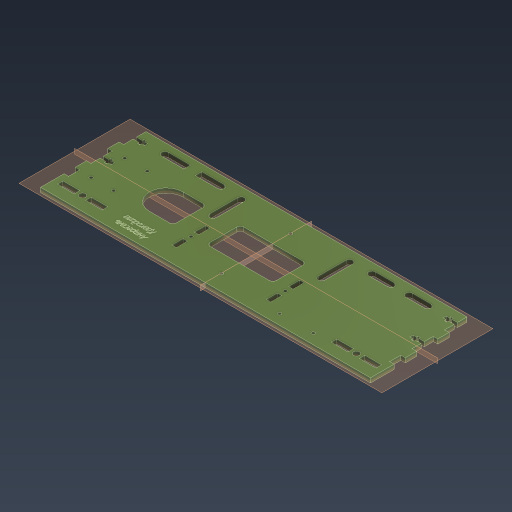
# Autodesk Inventor part: Фанерка_аккумуляторов
Saved by Autodesk Inventor 2023.2 (Build 272271030, 271C)
## iProperties
Created: 2025-12-29
Part Number: Фанерка_аккумуляторов
Material: Типовые
Document SubType Name: Modeling
Designer: Олег Коноваленко
Density: 1 g/cm^3
Appearance: Темно-оливковый
Author: Олег Коноваленко
Autodesk Inventor part; units mm, degrees
sketch "Эскиз1" plane through (0, 0, 0) normal (0, 1, 0) x (-1, 0, 0)
  line L0 (147, 45) -> (-147, 45)
  line L1 (-147, 45) -> (-147, -45)
  line L2 (-147, -45) -> (147, -45)
  line L3 (147, -45) -> (147, 45)
  line L4 (147, 45) -> (-147, -45) construction
  line L5 (-147, 45) -> (147, -45) construction
  point P0 (0, 0)
  dimension "d3" = 294
  dimension "d4" = 90
  constraints: 12 end point, 2 midpoint, 2 parallel, 1 horizontal, 1 perpendicular
  measures "d3" distance of L1.end L2.end
  measures "d4" distance of L0.end L1.end
extrude "Выдавливание1" add sketch "Эскиз1" along normal mid plane 4
sketch "Эскиз2" plane through (0, 2, 0) normal (0, 1, 0) x (1, 0, 0)
  line L0 (-127, -35) -> (-127, -30) projected
  line L1 (-127, -30) -> (-142, -30) projected
  line L2 (-142, -30) -> (-142, -35) projected
  line L3 (-142, -35) -> (-127, -35) projected
  line L4 (-102, -35) -> (-102, -30) projected
  line L5 (-102, -30) -> (-117, -30) projected
  line L6 (-117, -30) -> (-117, -35) projected
  line L7 (-117, -35) -> (-102, -35) projected
  line L8 (102, -35) -> (102, -30) projected
  line L9 (117, -35) -> (102, -35) projected
  line L10 (117, -30) -> (117, -35) projected
  line L11 (102, -30) -> (117, -30) projected
  line L12 (127, -35) -> (127, -30) projected
  line L13 (142, -35) -> (127, -35) projected
  line L14 (142, -30) -> (142, -35) projected
  line L15 (127, -30) -> (142, -30) projected
  circle A0 centre (122, -32.5) radius 2.8 projected
  circle A1 centre (-122, -32.5) radius 2.8 projected
  point P0 (0, 0)
extrude "Выдавливание2" cut sketch "Эскиз2" against normal up to next
sketch "Эскиз3" plane through (0, 2, 0) normal (0, 1, 0) x (1, 0, 0)
  line L0 (80, 0) -> (-80, 0) construction
  line L1 (80, 15) -> (-80, 15)
  line L2 (-80, -15) -> (80, -15)
  arc A0 (80, -15) -> (80, 15) centre (80, 0) ccw
  arc A1 (-80, 15) -> (-80, -15) centre (-80, 0) ccw
  line L3 (55, -15) -> (30, -15)
  line L4 (30, -15) -> (30, 15)
  line L5 (30, 15) -> (55, 15)
  line L6 (55, 15) -> (55, -15)
  line L7 (-29, -15) -> (-59, -15)
  line L8 (-59, -15) -> (-59, 15)
  line L9 (-59, 15) -> (-29, 15)
  line L10 (-29, 15) -> (-29, -15)
  line L11 (-44, -11) -> (-44, -1) projected
  line L12 (40, -11) -> (40, -1) projected
  point P0 (0, 0)
  point P1 (-29, 15)
  dimension "d7" = 160
  dimension "d8" = 15
  dimension "d11" = 25
  dimension "d12" = 30
  dimension "d13" = 10
  dimension "d14" = 15
  constraints: 24 end point, 5 parallel, 4 point on circle, 4 point on line, 4 tangent, 3 horizontal, 2 centre point, 2 perpendicular, 1 midpoint
  measures "d7" distance of L0.start L0.end
  measures "d8" distance between parallel lines of L2 L0
  measures "d11" distance between parallel lines of L4 L6
  measures "d12" distance between parallel lines of L8 L10
  measures "d13" distance between parallel lines of L4 L12
  measures "d14" distance between parallel lines of L8 L11
extrude "Выдавливание3" cut sketch "Эскиз3" against normal up to next contours L4 L2 L10 L1 | L8 L2 A1 L1
sketch "Эскиз4" plane through (0, 2, 0) normal (0, 1, 0) x (1, 0, 0)
  line L0 (40, -21) -> (44, -21) projected
  line L1 (44, -21) -> (44, -31) projected
  line L2 (40, -31) -> (40, -21) projected
  line L3 (40, -31) -> (44, -31) projected
  line L4 (44, -11) -> (40, -11) projected
  line L5 (44, -1) -> (44, -11) projected
  line L6 (40, -1) -> (44, -1) projected
  line L7 (40, -11) -> (40, -1) projected
  line L8 (-44, -21) -> (-40, -21) projected
  line L9 (-44, -31) -> (-44, -21) projected
  line L10 (-44, -31) -> (-40, -31) projected
  line L11 (-40, -21) -> (-40, -31) projected
  line L12 (-40, -11) -> (-44, -11) projected
  line L13 (-40, -1) -> (-40, -11) projected
  line L14 (-44, -1) -> (-40, -1) projected
  line L15 (-44, -11) -> (-44, -1) projected
  circle A0 centre (42, -16) radius 1.5
  circle A1 centre (-42, -16) radius 1.5
  line L16 (-42, 24.8) -> (-42, -50.8) construction
  line L17 (42, 24.8) -> (42, -50.8) construction
  point P0 (0, 0)
  dimension "d15" = 3
  dimension "d16" = 5
  dimension "d17" = 5
  constraints: 4 end point, 2 centre point, 2 point on line, 2 vertical, 1 equal radius, 4 other
  measures "d15" diameter of A1
  measures "d16" distance from line of L8 A1.centre
  measures "d17" distance from line of L0 A0.centre
extrude "Выдавливание4" cut sketch "Эскиз4" against normal up to next
fillet "Сопряжение1" radius 3 8 edges at (-29, 0, 15) (-29, 0, -15) (30, 0, -15) (30, 0, 15) (-59, 0, 15) (-59, 0, -15) (147, 0, -45) (-147, 0, -45)
sketch "Эскиз6" plane through (0, 2, 0) normal (0, 1, 0) x (1, 0, 0)
  line L0 (117.25, 36) -> (67.25, 36) construction
  line L1 (117.25, 39) -> (67.25, 39)
  line L2 (67.25, 33) -> (117.25, 33)
  arc A0 (117.25, 33) -> (117.25, 39) centre (117.25, 36) ccw
  arc A1 (67.25, 39) -> (67.25, 33) centre (67.25, 36) ccw
  line L3 (144, 45) -> (-144, 45) projected
  line L4 (0, 63) -> (0, -63) projected
  line L5 (147, -45) -> (147, 42) projected
  line L6 (97.25, 33) -> (97.25, 39)
  line L7 (87.25, 33) -> (87.25, 39)
  line L8 (97.25, 36) -> (87.25, 36) construction
  point P0 (0, 0)
  point P1 (92.25, 36)
  point P2 (92.25, 36)
  dimension "d23" = 9
  dimension "d24" = 50
  dimension "d26" = 3
  dimension "d29" = 54.75
  dimension "d30" = 10
  constraints: 14 end point, 4 midpoint, 4 point on circle, 4 point on line, 4 tangent, 2 centre point, 2 perpendicular, 1 coincident, 1 horizontal, 1 parallel
  measures "d23" distance from line of L3 point (92.25, 36)
  measures "d24" distance of L0.start L0.end
  measures "d26" distance between parallel lines of L2 L0
  measures "d29" distance from line of L5 point (92.25, 36)
  measures "d30" distance of L8.start L8.end
extrude "Выдавливание6" cut sketch "Эскиз6" against normal up to next contours A0 L2 L6 L1 | L7 L2 A1 L1
fillet "Сопряжение2" radius 3 4 edges at (97.25, 0, -33) (97.25, 0, -39) (87.25, 0, -39) (87.25, 0, -33)
mirror "Зеркальное отражение1" about plane through (0, 0, 0) normal (1, 0, 0) of "Выдавливание6"
sketch "Эскиз7" plane through (0, 2, 0) normal (0, 1, 0) x (1, 0, 0)
  line L0 (-48.25, 10) -> (-48.25, 35) construction
  line L1 (-45.25, 10) -> (-45.25, 35)
  line L2 (-51.25, 35) -> (-51.25, 10)
  arc A0 (-51.25, 10) -> (-45.25, 10) centre (-48.25, 10) ccw
  arc A1 (-45.25, 35) -> (-51.25, 35) centre (-48.25, 35) ccw
  line L3 (144, 45) -> (-144, 45) projected
  line L4 (-59, 12) -> (-59, -12) projected
  line L5 (-37.5, 4) -> (-37.5, 0.5) projected
  point P0 (0, 0)
  point P1 (-48.25, 22.5)
  dimension "d32" = 3
  dimension "d33" = 25
  dimension "d34" = 22.5
  dimension "d35" = 10.75
  constraints: 8 end point, 4 point on circle, 4 tangent, 2 centre point, 1 midpoint, 1 parallel, 1 vertical
  measures "d32" distance between parallel lines of L2 L0
  measures "d33" distance of L0.start L0.end
  measures "d34" distance from line of L3 point (-48.25, 22.5)
  measures "d35" distance from line of L4 point (-48.25, 22.5)
extrude "Выдавливание7" cut sketch "Эскиз7" against normal up to next
sketch "Эскиз8" plane through (0, 2, 0) normal (0, 1, 0) x (1, 0, 0)
  spline S0 degree 3 poles (0.1, -29.25) (-0.0887, -29.25) (-0.2898, -29.2878) (-0.6592, -29.441) (-0.8277, -29.5564) (-1.0936, -29.8223) (-1.209, -29.9908) (-1.3622, -30.3602) (-1.4, -30.5613) (-1.4, -30.9387) (-1.3622, -31.1398) (-1.209, -31.5092) (-1.0936, -31.6777) (-0.8277, -31.9436) (-0.6592, -32.059) (-0.2898, -32.2122) (-0.0887, -32.25) (0.2887, -32.25) (0.4898, -32.2122) (0.8592, -32.059) (1.0277, -31.9436) (1.2936, -31.6777) (1.409, -31.5092) (1.5622, -31.1398) (1.6, -30.9387) (1.6, -30.5613) (1.5622, -30.3602) (1.409, -29.9908) (1.2936, -29.8223) (1.0277, -29.5564) (0.8592, -29.441) (0.4898, -29.2878) (0.2887, -29.25) (0.1, -29.25) knots -0.905867 -0.905867 -0.905867 -0.905867 -0.84925 -0.84925 -0.792632 -0.792632 -0.736016 -0.736016 -0.6794 -0.6794 -0.622784 -0.622784 -0.566168 -0.566168 -0.509551 -0.509551 -0.452934 -0.452934 -0.396316 -0.396316 -0.339699 -0.339699 -0.283083 -0.283083 -0.226467 -0.226467 -0.169851 -0.169851 -0.113235 -0.113235 -0.056617 -0.056617 0 0 0 0 projected
  spline S1 degree 3 poles (0.1, 32.25) (-0.0887, 32.25) (-0.2898, 32.2122) (-0.6592, 32.059) (-0.8277, 31.9436) (-1.0936, 31.6777) (-1.209, 31.5092) (-1.3622, 31.1398) (-1.4, 30.9387) (-1.4, 30.5613) (-1.3622, 30.3602) (-1.209, 29.9908) (-1.0936, 29.8223) (-0.8277, 29.5564) (-0.6592, 29.441) (-0.2898, 29.2878) (-0.0887, 29.25) (0.2887, 29.25) (0.4898, 29.2878) (0.8592, 29.441) (1.0277, 29.5564) (1.2936, 29.8223) (1.409, 29.9908) (1.5622, 30.3602) (1.6, 30.5613) (1.6, 30.9387) (1.5622, 31.1398) (1.409, 31.5092) (1.2936, 31.6777) (1.0277, 31.9436) (0.8592, 32.059) (0.4898, 32.2122) (0.2887, 32.25) (0.1, 32.25) knots -0.905867 -0.905867 -0.905867 -0.905867 -0.84925 -0.84925 -0.792632 -0.792632 -0.736016 -0.736016 -0.6794 -0.6794 -0.622784 -0.622784 -0.566168 -0.566168 -0.509551 -0.509551 -0.452934 -0.452934 -0.396316 -0.396316 -0.339699 -0.339699 -0.283083 -0.283083 -0.226467 -0.226467 -0.169851 -0.169851 -0.113235 -0.113235 -0.056617 -0.056617 0 0 0 0 projected
  point P0 (0, 0)
  point P1 (0.1, -29.25)
  point P2 (0.1, 32.25)
extrude "Выдавливание8" cut sketch "Эскиз8" against normal up to next
mirror "Зеркальное отражение2" about plane through (0, 0, 0) normal (1, 0, 0) of "Выдавливание7"
sketch "Эскиз9" plane through (0, 2, 0) normal (0, 1, 0) x (1, 0, 0)
  line L0 (-53.0582, -40.3435) -> (-94.511, -40.3435) construction
  line L1 (-94.511, -40.3435) -> (-94.511, -22.9258) construction
  line L2 (-94.511, -22.9258) -> (-53.0582, -22.9258) construction
  line L3 (-53.0582, -22.9258) -> (-53.0582, -40.3435) construction
  line L4 (-61.6229, -36.7976) -> (-60.8336, -35.5068)
  spline S0 degree 2 poles (-60.8336, -35.5068) (-60.752, -35.3746) (-60.6237, -35.3746) knots 0 0 0 1 1 1
  spline S1 degree 2 poles (-60.6237, -35.3746) (-60.4409, -35.3746) (-60.4992, -35.5457) knots 0 0 0 1 1 1
  spline S2 degree 2 poles (-60.4992, -35.5457) (-60.507, -35.569) (-60.5226, -35.6001) knots 0 0 0 1 1 1
  line L5 (-60.5226, -35.6001) -> (-63.3258, -40.1841)
  spline S3 degree 2 poles (-63.3258, -40.1841) (-63.423, -40.3435) (-63.5513, -40.3435) knots 0 0 0 1 1 1
  spline S4 degree 2 poles (-63.5513, -40.3435) (-63.6796, -40.3435) (-63.668, -40.1841) knots 0 0 0 1 1 1
  line L6 (-63.668, -40.1841) -> (-63.3531, -35.6001)
  spline S5 degree 2 poles (-63.3531, -35.6001) (-63.3531, -35.569) (-63.3453, -35.5457) knots 0 0 0 1 1 1
  spline S6 degree 2 poles (-63.3453, -35.5457) (-63.287, -35.3746) (-63.1042, -35.3746) knots 0 0 0 1 1 1
  spline S7 degree 2 poles (-63.1042, -35.3746) (-62.972, -35.3746) (-62.9798, -35.5068) knots 0 0 0 1 1 1
  line L7 (-62.9798, -35.5068) -> (-63.0731, -36.7976)
  line L8 (-63.0731, -36.7976) -> (-61.6229, -36.7976)
  line L9 (-63.0964, -37.1514) -> (-63.2636, -39.4959)
  line L10 (-63.2636, -39.4959) -> (-61.8367, -37.1514)
  line L11 (-61.8367, -37.1514) -> (-63.0964, -37.1514)
  spline S8 degree 2 poles (-66.203, -35.5496) (-66.1408, -35.3707) (-65.9658, -35.3707) knots 0 0 0 1 1 1
  spline S9 degree 2 poles (-65.9658, -35.3707) (-65.787, -35.3707) (-65.8492, -35.5496) knots 0 0 0 1 1 1
  line L12 (-65.8492, -35.5496) -> (-66.3313, -36.9726)
  line L13 (-66.3313, -36.9726) -> (-64.9005, -36.9726)
  line L14 (-64.9005, -36.9726) -> (-64.4184, -35.5496)
  spline S10 degree 2 poles (-64.4184, -35.5496) (-64.3562, -35.3707) (-64.1812, -35.3707) knots 0 0 0 1 1 1
  spline S11 degree 2 poles (-64.1812, -35.3707) (-64.0024, -35.3707) (-64.0646, -35.5496) knots 0 0 0 1 1 1
  line L15 (-64.0646, -35.5496) -> (-65.1493, -38.7494)
  spline S12 degree 2 poles (-65.1493, -38.7494) (-65.2115, -38.9283) (-65.3865, -38.9283) knots 0 0 0 1 1 1
  spline S13 degree 2 poles (-65.3865, -38.9283) (-65.5653, -38.9283) (-65.5031, -38.7494) knots 0 0 0 1 1 1
  line L16 (-65.5031, -38.7494) -> (-65.021, -37.3264)
  line L17 (-65.021, -37.3264) -> (-66.4518, -37.3264)
  line L18 (-66.4518, -37.3264) -> (-66.9339, -38.7494)
  spline S14 degree 2 poles (-66.9339, -38.7494) (-66.9961, -38.9283) (-67.1711, -38.9283) knots 0 0 0 1 1 1
  spline S15 degree 2 poles (-67.1711, -38.9283) (-67.3499, -38.9283) (-67.2877, -38.7494) knots 0 0 0 1 1 1
  line L19 (-67.2877, -38.7494) -> (-66.203, -35.5496)
  line L20 (-69.3601, -38.5744) -> (-68.2908, -38.5744)
  line L21 (-68.2908, -38.5744) -> (-67.2644, -35.5496)
  spline S16 degree 2 poles (-67.2644, -35.5496) (-67.2022, -35.3707) (-67.0272, -35.3707) knots 0 0 0 1 1 1
  spline S17 degree 2 poles (-67.0272, -35.3707) (-66.8484, -35.3707) (-66.9106, -35.5496) knots 0 0 0 1 1 1
  line L22 (-66.9106, -35.5496) -> (-67.9954, -38.7494)
  spline S18 degree 2 poles (-67.9954, -38.7494) (-68.0576, -38.9283) (-68.2364, -38.9283) knots 0 0 0 1 1 1
  line L23 (-68.2364, -38.9283) -> (-70.5459, -38.9283)
  spline S19 degree 2 poles (-70.5459, -38.9283) (-70.8375, -38.9283) (-71.1136, -38.5083) (-71.0164, -38.2167) knots 0 0 0 1 2 2 2
  line L24 (-71.0164, -38.2167) -> (-70.1104, -35.5496)
  spline S20 degree 2 poles (-70.1104, -35.5496) (-70.0482, -35.3707) (-69.8733, -35.3707) knots 0 0 0 1 1 1
  spline S21 degree 2 poles (-69.8733, -35.3707) (-69.6944, -35.3707) (-69.7566, -35.5496) knots 0 0 0 1 1 1
  line L25 (-69.7566, -35.5496) -> (-70.6625, -38.2167)
  spline S22 degree 2 poles (-70.6625, -38.2167) (-70.7131, -38.3645) (-70.5731, -38.5744) (-70.4254, -38.5744) knots 0 0 0 1 2 2 2
  line L26 (-70.4254, -38.5744) -> (-69.7139, -38.5744)
  line L27 (-69.7139, -38.5744) -> (-68.6874, -35.5496)
  spline S23 degree 2 poles (-68.6874, -35.5496) (-68.6252, -35.3707) (-68.4503, -35.3707) knots 0 0 0 1 1 1
  spline S24 degree 2 poles (-68.4503, -35.3707) (-68.2714, -35.3707) (-68.3336, -35.5496) knots 0 0 0 1 1 1
  line L28 (-68.3336, -35.5496) -> (-69.3601, -38.5744)
  line L29 (-71.1097, -35.3668) -> (-70.6859, -34.1265)
  spline S25 degree 2 poles (-70.6859, -34.1265) (-70.6275, -33.9477) (-70.4487, -33.9477) knots 0 0 0 1 1 1
  spline S26 degree 2 poles (-70.4487, -33.9477) (-70.2737, -33.9477) (-70.3321, -34.1265) knots 0 0 0 1 1 1
  line L30 (-70.3321, -34.1265) -> (-71.9028, -38.7494)
  spline S27 degree 2 poles (-71.9028, -38.7494) (-71.965, -38.9283) (-72.1439, -38.9283) knots 0 0 0 1 1 1
  line L31 (-72.1439, -38.9283) -> (-73.3958, -38.9283)
  spline S28 degree 2 poles (-73.3958, -38.9283) (-73.6874, -38.9283) (-73.9635, -38.5122) (-73.8624, -38.2206) knots 0 0 0 1 2 2 2
  line L32 (-73.8624, -38.2206) -> (-73.1353, -36.0822)
  spline S29 degree 2 poles (-73.1353, -36.0822) (-73.0381, -35.7906) (-72.4744, -35.3668) (-72.1828, -35.3668) knots 0 0 0 1 2 2 2
  line L33 (-72.1828, -35.3668) -> (-71.1097, -35.3668)
  line L34 (-71.2302, -35.7206) -> (-72.3072, -35.7206)
  spline S30 degree 2 poles (-72.3072, -35.7206) (-72.451, -35.7206) (-72.731, -35.9345) (-72.7815, -36.0822) knots 0 0 0 1 2 2 2
  line L35 (-72.7815, -36.0822) -> (-73.5086, -38.2206)
  spline S31 degree 2 poles (-73.5086, -38.2206) (-73.5591, -38.3645) (-73.4192, -38.5744) (-73.2753, -38.5744) knots 0 0 0 1 2 2 2
  line L36 (-73.2753, -38.5744) -> (-72.1983, -38.5744)
  line L37 (-72.1983, -38.5744) -> (-71.2302, -35.7206)
  line L38 (-74.5, -36.9687) -> (-74.1968, -36.0783)
  spline S32 degree 2 poles (-74.1968, -36.0783) (-74.1462, -35.9345) (-74.2823, -35.7245) (-74.43, -35.7245) knots 0 0 0 1 2 2 2
  line L39 (-74.43, -35.7245) -> (-75.6781, -35.7245)
  spline S33 degree 2 poles (-75.6781, -35.7245) (-75.8569, -35.7245) (-75.7947, -35.5496) knots 0 0 0 1 1 1
  spline S34 degree 2 poles (-75.7947, -35.5496) (-75.7364, -35.3707) (-75.5576, -35.3707) knots 0 0 0 1 1 1
  line L40 (-75.5576, -35.3707) -> (-74.3095, -35.3707)
  spline S35 degree 2 poles (-74.3095, -35.3707) (-74.014, -35.3707) (-73.7419, -35.7867) (-73.8429, -36.0822) knots 0 0 0 1 2 2 2
  line L41 (-73.8429, -36.0822) -> (-74.5661, -38.209)
  spline S36 degree 2 poles (-74.5661, -38.209) (-74.6672, -38.5006) (-75.2271, -38.9205) (-75.5187, -38.9205) knots 0 0 0 1 2 2 2
  line L42 (-75.5187, -38.9205) -> (-76.2341, -38.9205)
  spline S37 degree 2 poles (-76.2341, -38.9205) (-76.5296, -38.9205) (-76.8056, -38.5045) (-76.7045, -38.209) knots 0 0 0 1 2 2 2
  line L43 (-76.7045, -38.209) -> (-76.3429, -37.1475)
  spline S38 degree 2 poles (-76.3429, -37.1475) (-76.2846, -36.9687) (-76.1019, -36.9687) knots 0 0 0 1 1 1
  line L44 (-76.1019, -36.9687) -> (-74.5, -36.9687)
  line L45 (-74.6205, -37.3225) -> (-76.0513, -37.3225)
  line L46 (-76.0513, -37.3225) -> (-76.3507, -38.2129)
  spline S39 degree 2 poles (-76.3507, -38.2129) (-76.4013, -38.3567) (-76.2613, -38.5667) (-76.1136, -38.5667) knots 0 0 0 1 2 2 2
  line L47 (-76.1136, -38.5667) -> (-75.3943, -38.5667)
  spline S40 degree 2 poles (-75.3943, -38.5667) (-75.2504, -38.5667) (-74.9705, -38.3567) (-74.9199, -38.2129) knots 0 0 0 1 2 2 2
  line L48 (-74.9199, -38.2129) -> (-74.6205, -37.3225)
  line L49 (-78.4075, -35.3707) -> (-77.1594, -35.3707)
  spline S41 degree 2 poles (-77.1594, -35.3707) (-76.8678, -35.3707) (-76.5918, -35.7867) (-76.6929, -36.0822) knots 0 0 0 1 2 2 2
  line L50 (-76.6929, -36.0822) -> (-77.4199, -38.2167)
  spline S42 degree 2 poles (-77.4199, -38.2167) (-77.5171, -38.5083) (-78.077, -38.9283) (-78.3686, -38.9283) knots 0 0 0 1 2 2 2
  line L51 (-78.3686, -38.9283) -> (-79.6167, -38.9283)
  spline S43 degree 2 poles (-79.6167, -38.9283) (-79.7916, -38.9283) (-79.7333, -38.7533) knots 0 0 0 1 1 1
  spline S44 degree 2 poles (-79.7333, -38.7533) (-79.6711, -38.5744) (-79.4961, -38.5744) knots 0 0 0 1 1 1
  line L52 (-79.4961, -38.5744) -> (-78.2481, -38.5744)
  spline S45 degree 2 poles (-78.2481, -38.5744) (-78.1042, -38.5744) (-77.8243, -38.3645) (-77.7737, -38.2167) knots 0 0 0 1 2 2 2
  line L53 (-77.7737, -38.2167) -> (-77.0467, -36.0822)
  spline S46 degree 2 poles (-77.0467, -36.0822) (-76.9961, -35.9345) (-77.1361, -35.7245) (-77.28, -35.7245) knots 0 0 0 1 2 2 2
  line L54 (-77.28, -35.7245) -> (-78.5241, -35.7245)
  spline S47 degree 2 poles (-78.5241, -35.7245) (-78.703, -35.7245) (-78.6447, -35.5496) knots 0 0 0 1 1 1
  spline S48 degree 2 poles (-78.6447, -35.5496) (-78.5824, -35.3707) (-78.4075, -35.3707) knots 0 0 0 1 1 1
  spline S49 degree 2 poles (-81.6734, -36.0822) (-81.5723, -35.7867) (-81.0164, -35.3707) (-80.7209, -35.3707) knots 0 0 0 1 2 2 2
  line L55 (-80.7209, -35.3707) -> (-80.0055, -35.3707)
  spline S50 degree 2 poles (-80.0055, -35.3707) (-79.71, -35.3707) (-79.4339, -35.7867) (-79.535, -36.0822) knots 0 0 0 1 2 2 2
  line L56 (-79.535, -36.0822) -> (-80.2621, -38.2167)
  spline S51 degree 2 poles (-80.2621, -38.2167) (-80.3593, -38.5083) (-80.923, -38.9283) (-81.2146, -38.9283) knots 0 0 0 1 2 2 2
  line L57 (-81.2146, -38.9283) -> (-81.93, -38.9283)
  spline S52 degree 2 poles (-81.93, -38.9283) (-82.2216, -38.9283) (-82.4977, -38.5083) (-82.4005, -38.2167) knots 0 0 0 1 2 2 2
  line L58 (-82.4005, -38.2167) -> (-81.6734, -36.0822)
  line L59 (-81.3196, -36.0822) -> (-82.0467, -38.2167)
  spline S53 degree 2 poles (-82.0467, -38.2167) (-82.0972, -38.3645) (-81.9573, -38.5744) (-81.8095, -38.5744) knots 0 0 0 1 2 2 2
  line L60 (-81.8095, -38.5744) -> (-81.0941, -38.5744)
  spline S54 degree 2 poles (-81.0941, -38.5744) (-80.9464, -38.5744) (-80.6664, -38.3645) (-80.6159, -38.2167) knots 0 0 0 1 2 2 2
  line L61 (-80.6159, -38.2167) -> (-79.8888, -36.0822)
  spline S55 degree 2 poles (-79.8888, -36.0822) (-79.8383, -35.9345) (-79.9782, -35.7245) (-80.126, -35.7245) knots 0 0 0 1 2 2 2
  line L62 (-80.126, -35.7245) -> (-80.8414, -35.7245)
  spline S56 degree 2 poles (-80.8414, -35.7245) (-80.9891, -35.7245) (-81.2691, -35.9345) (-81.3196, -36.0822) knots 0 0 0 1 2 2 2
  spline S57 degree 2 poles (-84.3367, -35.5496) (-84.2745, -35.3707) (-84.0996, -35.3707) knots 0 0 0 1 1 1
  spline S58 degree 2 poles (-84.0996, -35.3707) (-83.9207, -35.3707) (-83.9829, -35.5496) knots 0 0 0 1 1 1
  line L63 (-83.9829, -35.5496) -> (-85.0094, -38.5744)
  line L64 (-85.0094, -38.5744) -> (-84.2629, -38.5744)
  line L65 (-84.2629, -38.5744) -> (-82.5405, -35.5107)
  spline S59 degree 2 poles (-82.5405, -35.5107) (-82.4627, -35.3707) (-82.3227, -35.3707) knots 0 0 0 1 1 1
  spline S60 degree 2 poles (-82.3227, -35.3707) (-82.1439, -35.3707) (-82.2022, -35.5418) knots 0 0 0 1 1 1
  spline S61 degree 2 poles (-82.2022, -35.5418) (-82.21, -35.5612) (-82.2216, -35.5884) knots 0 0 0 1 1 1
  line L66 (-82.2216, -35.5884) -> (-84.0179, -38.7883)
  spline S62 degree 2 poles (-84.0179, -38.7883) (-84.0996, -38.9283) (-84.2395, -38.9283) knots 0 0 0 1 1 1
  line L67 (-84.2395, -38.9283) -> (-85.3048, -38.9283)
  spline S63 degree 2 poles (-85.3048, -38.9283) (-85.4837, -38.9283) (-85.4215, -38.7494) knots 0 0 0 1 1 1
  line L68 (-85.4215, -38.7494) -> (-84.3367, -35.5496)
  spline S64 degree 2 poles (-87.3655, -36.0822) (-87.2644, -35.7867) (-86.7084, -35.3707) (-86.4129, -35.3707) knots 0 0 0 1 2 2 2
  line L69 (-86.4129, -35.3707) -> (-85.1649, -35.3707)
  spline S65 degree 2 poles (-85.1649, -35.3707) (-84.986, -35.3707) (-85.0482, -35.5496) knots 0 0 0 1 1 1
  line L70 (-85.0482, -35.5496) -> (-86.133, -38.7494)
  spline S66 degree 2 poles (-86.133, -38.7494) (-86.1952, -38.9283) (-86.3702, -38.9283) knots 0 0 0 1 1 1
  spline S67 degree 2 poles (-86.3702, -38.9283) (-86.549, -38.9283) (-86.4868, -38.7494) knots 0 0 0 1 1 1
  line L71 (-86.4868, -38.7494) -> (-86.0047, -37.3264)
  line L72 (-86.0047, -37.3264) -> (-87.0739, -37.3264)
  spline S68 degree 2 poles (-87.0739, -37.3264) (-87.3733, -37.3264) (-87.6454, -36.9065) (-87.5482, -36.6149) knots 0 0 0 1 2 2 2
  line L73 (-87.5482, -36.6149) -> (-87.3655, -36.0822)
  line L74 (-87.0117, -36.0822) -> (-87.1944, -36.6149)
  spline S69 degree 2 poles (-87.1944, -36.6149) (-87.245, -36.7626) (-87.105, -36.9726) (-86.9573, -36.9726) knots 0 0 0 1 2 2 2
  line L75 (-86.9573, -36.9726) -> (-85.8842, -36.9726)
  line L76 (-85.8842, -36.9726) -> (-85.4604, -35.7245)
  line L77 (-85.4604, -35.7245) -> (-86.5335, -35.7245)
  spline S70 degree 2 poles (-86.5335, -35.7245) (-86.6812, -35.7245) (-86.9611, -35.9345) (-87.0117, -36.0822) knots 0 0 0 1 2 2 2
  line L78 (-61.9786, -29.5483) -> (-61.3954, -27.8298)
  spline S71 degree 2 poles (-61.3954, -27.8298) (-61.3332, -27.651) (-61.1583, -27.651) knots 0 0 0 1 1 1
  spline S72 degree 2 poles (-61.1583, -27.651) (-60.9794, -27.651) (-61.0416, -27.8298) knots 0 0 0 1 1 1
  line L79 (-61.0416, -27.8298) -> (-62.6085, -32.4488)
  spline S73 degree 2 poles (-62.6085, -32.4488) (-62.6707, -32.6276) (-62.8496, -32.6276) knots 0 0 0 1 1 1
  spline S74 degree 2 poles (-62.8496, -32.6276) (-63.0245, -32.6276) (-62.9623, -32.4488) knots 0 0 0 1 1 1
  line L80 (-62.9623, -32.4488) -> (-62.1808, -30.1432)
  line L81 (-62.1808, -30.1432) -> (-64.8169, -32.5576)
  spline S75 degree 2 poles (-64.8169, -32.5576) (-64.8947, -32.6315) (-64.9802, -32.6315) knots 0 0 0 1 1 1
  spline S76 degree 2 poles (-64.9802, -32.6315) (-65.0541, -32.6315) (-65.1279, -32.5227) (-65.1046, -32.4488) knots 0 0 0 1 2 2 2
  spline S77 degree 2 poles (-65.1046, -32.4488) (-65.0852, -32.3943) (-65.0307, -32.3438) knots 0 0 0 1 1 1
  line L82 (-65.0307, -32.3438) -> (-63.1917, -30.6603)
  line L83 (-63.1917, -30.6603) -> (-63.5377, -27.9037)
  spline S78 degree 2 poles (-63.5377, -27.9037) (-63.5416, -27.8648) (-63.53, -27.822) knots 0 0 0 1 1 1
  spline S79 degree 2 poles (-63.53, -27.822) (-63.4716, -27.651) (-63.285, -27.651) knots 0 0 0 1 1 1
  spline S80 degree 2 poles (-63.285, -27.651) (-63.1839, -27.651) (-63.1684, -27.7559) knots 0 0 0 1 1 1
  line L84 (-63.1684, -27.7559) -> (-62.8418, -30.3415)
  line L85 (-62.8418, -30.3415) -> (-61.9786, -29.5483)
  line L86 (-64.5292, -27.6471) -> (-64.1054, -26.4068)
  spline S81 degree 2 poles (-64.1054, -26.4068) (-64.0471, -26.2279) (-63.8682, -26.2279) knots 0 0 0 1 1 1
  spline S82 degree 2 poles (-63.8682, -26.2279) (-63.6933, -26.2279) (-63.7516, -26.4068) knots 0 0 0 1 1 1
  line L87 (-63.7516, -26.4068) -> (-65.3223, -31.0297)
  spline S83 degree 2 poles (-65.3223, -31.0297) (-65.3845, -31.2085) (-65.5634, -31.2085) knots 0 0 0 1 1 1
  line L88 (-65.5634, -31.2085) -> (-66.8153, -31.2085)
  spline S84 degree 2 poles (-66.8153, -31.2085) (-67.1069, -31.2085) (-67.383, -30.7925) (-67.2819, -30.5009) knots 0 0 0 1 2 2 2
  line L89 (-67.2819, -30.5009) -> (-66.5548, -28.3625)
  spline S85 degree 2 poles (-66.5548, -28.3625) (-66.4576, -28.0709) (-65.8939, -27.6471) (-65.6023, -27.6471) knots 0 0 0 1 2 2 2
  line L90 (-65.6023, -27.6471) -> (-64.5292, -27.6471)
  line L91 (-64.6497, -28.0009) -> (-65.7267, -28.0009)
  spline S86 degree 2 poles (-65.7267, -28.0009) (-65.8705, -28.0009) (-66.1505, -28.2147) (-66.201, -28.3625) knots 0 0 0 1 2 2 2
  line L92 (-66.201, -28.3625) -> (-66.9281, -30.5009)
  spline S87 degree 2 poles (-66.9281, -30.5009) (-66.9786, -30.6447) (-66.8387, -30.8547) (-66.6948, -30.8547) knots 0 0 0 1 2 2 2
  line L93 (-66.6948, -30.8547) -> (-65.6178, -30.8547)
  line L94 (-65.6178, -30.8547) -> (-64.6497, -28.0009)
  spline S88 degree 2 poles (-69.4009, -28.3625) (-69.2998, -28.067) (-68.7438, -27.651) (-68.4483, -27.651) knots 0 0 0 1 2 2 2
  line L95 (-68.4483, -27.651) -> (-67.7329, -27.651)
  spline S89 degree 2 poles (-67.7329, -27.651) (-67.4374, -27.651) (-67.1614, -28.067) (-67.2625, -28.3625) knots 0 0 0 1 2 2 2
  line L96 (-67.2625, -28.3625) -> (-67.9895, -30.497)
  spline S90 degree 2 poles (-67.9895, -30.497) (-68.0867, -30.7886) (-68.6505, -31.2085) (-68.9421, -31.2085) knots 0 0 0 1 2 2 2
  line L97 (-68.9421, -31.2085) -> (-69.6575, -31.2085)
  spline S91 degree 2 poles (-69.6575, -31.2085) (-69.9491, -31.2085) (-70.2251, -30.7886) (-70.1279, -30.497) knots 0 0 0 1 2 2 2
  line L98 (-70.1279, -30.497) -> (-69.4009, -28.3625)
  line L99 (-69.0471, -28.3625) -> (-69.7741, -30.497)
  spline S92 degree 2 poles (-69.7741, -30.497) (-69.8247, -30.6447) (-69.6847, -30.8547) (-69.537, -30.8547) knots 0 0 0 1 2 2 2
  line L100 (-69.537, -30.8547) -> (-68.8216, -30.8547)
  spline S93 degree 2 poles (-68.8216, -30.8547) (-68.6738, -30.8547) (-68.3939, -30.6447) (-68.3433, -30.497) knots 0 0 0 1 2 2 2
  line L101 (-68.3433, -30.497) -> (-67.6163, -28.3625)
  spline S94 degree 2 poles (-67.6163, -28.3625) (-67.5657, -28.2147) (-67.7057, -28.0048) (-67.8534, -28.0048) knots 0 0 0 1 2 2 2
  line L102 (-67.8534, -28.0048) -> (-68.5688, -28.0048)
  spline S95 degree 2 poles (-68.5688, -28.0048) (-68.7166, -28.0048) (-68.9965, -28.2147) (-69.0471, -28.3625) knots 0 0 0 1 2 2 2
  spline S96 degree 2 poles (-73.1567, -31.0141) (-73.1373, -30.9519) (-73.0673, -30.8936) knots 0 0 0 1 1 1
  spline S97 degree 2 poles (-73.0673, -30.8936) (-72.3091, -30.2909) (-71.5548, -29.6883) knots 0 0 0 1 1 1
  line L103 (-71.5548, -29.6883) -> (-72.0719, -27.9231)
  spline S98 degree 2 poles (-72.0719, -27.9231) (-72.0836, -27.8804) (-72.0681, -27.8298) knots 0 0 0 1 1 1
  spline S99 degree 2 poles (-72.0681, -27.8298) (-72.0408, -27.7559) (-71.8931, -27.651) (-71.8231, -27.651) knots 0 0 0 1 2 2 2
  spline S100 degree 2 poles (-71.8231, -27.651) (-71.7337, -27.651) (-71.7065, -27.7326) knots 0 0 0 1 1 1
  line L104 (-71.7065, -27.7326) -> (-71.2166, -29.4161)
  spline S101 degree 2 poles (-71.2166, -29.4161) (-71.0727, -29.2995) (-70.6839, -28.9845) knots 0 0 0 1 1 1
  line L105 (-70.6839, -28.9845) -> (-70.2912, -27.8298)
  spline S102 degree 2 poles (-70.2912, -27.8298) (-70.229, -27.651) (-70.0541, -27.651) knots 0 0 0 1 1 1
  spline S103 degree 2 poles (-70.0541, -27.651) (-69.8752, -27.651) (-69.9374, -27.8298) knots 0 0 0 1 1 1
  line L106 (-69.9374, -27.8298) -> (-71.0222, -31.0297)
  spline S104 degree 2 poles (-71.0222, -31.0297) (-71.0844, -31.2085) (-71.2594, -31.2085) knots 0 0 0 1 1 1
  spline S105 degree 2 poles (-71.2594, -31.2085) (-71.4382, -31.2085) (-71.376, -31.0297) knots 0 0 0 1 1 1
  line L107 (-71.376, -31.0297) -> (-70.8628, -29.5172)
  line L108 (-70.8628, -29.5172) -> (-72.8845, -31.1346)
  spline S106 degree 2 poles (-72.8845, -31.1346) (-72.9623, -31.1968) (-73.0323, -31.1968) knots 0 0 0 1 1 1
  spline S107 degree 2 poles (-73.0323, -31.1968) (-73.1101, -31.1968) (-73.18, -31.088) (-73.1567, -31.0141) knots 0 0 0 1 2 2 2
  spline S108 degree 2 poles (-75.0929, -28.3625) (-74.9919, -28.067) (-74.4359, -27.651) (-74.1404, -27.651) knots 0 0 0 1 2 2 2
  line L109 (-74.1404, -27.651) -> (-73.425, -27.651)
  spline S109 degree 2 poles (-73.425, -27.651) (-73.1295, -27.651) (-72.8534, -28.067) (-72.9545, -28.3625) knots 0 0 0 1 2 2 2
  line L110 (-72.9545, -28.3625) -> (-73.6816, -30.497)
  spline S110 degree 2 poles (-73.6816, -30.497) (-73.7788, -30.7886) (-74.3426, -31.2085) (-74.6342, -31.2085) knots 0 0 0 1 2 2 2
  line L111 (-74.6342, -31.2085) -> (-75.3496, -31.2085)
  spline S111 degree 2 poles (-75.3496, -31.2085) (-75.6412, -31.2085) (-75.9172, -30.7886) (-75.82, -30.497) knots 0 0 0 1 2 2 2
  line L112 (-75.82, -30.497) -> (-75.0929, -28.3625)
  line L113 (-74.7391, -28.3625) -> (-75.4662, -30.497)
  spline S112 degree 2 poles (-75.4662, -30.497) (-75.5167, -30.6447) (-75.3768, -30.8547) (-75.229, -30.8547) knots 0 0 0 1 2 2 2
  line L114 (-75.229, -30.8547) -> (-74.5136, -30.8547)
  spline S113 degree 2 poles (-74.5136, -30.8547) (-74.3659, -30.8547) (-74.0859, -30.6447) (-74.0354, -30.497) knots 0 0 0 1 2 2 2
  line L115 (-74.0354, -30.497) -> (-73.3083, -28.3625)
  spline S114 degree 2 poles (-73.3083, -28.3625) (-73.2578, -28.2147) (-73.3978, -28.0048) (-73.5455, -28.0048) knots 0 0 0 1 2 2 2
  line L116 (-73.5455, -28.0048) -> (-74.2609, -28.0048)
  spline S115 degree 2 poles (-74.2609, -28.0048) (-74.4087, -28.0048) (-74.6886, -28.2147) (-74.7391, -28.3625) knots 0 0 0 1 2 2 2
  spline S116 degree 2 poles (-77.939, -28.3625) (-77.8418, -28.0709) (-77.2819, -27.651) (-76.9825, -27.651) knots 0 0 0 1 2 2 2
  line L117 (-76.9825, -27.651) -> (-76.2749, -27.651)
  spline S117 degree 2 poles (-76.2749, -27.651) (-75.9755, -27.651) (-75.7034, -28.0709) (-75.8006, -28.3625) knots 0 0 0 1 2 2 2
  line L118 (-75.8006, -28.3625) -> (-76.5276, -30.497)
  spline S118 degree 2 poles (-76.5276, -30.497) (-76.6287, -30.7925) (-77.1847, -31.2085) (-77.4841, -31.2085) knots 0 0 0 1 2 2 2
  line L119 (-77.4841, -31.2085) -> (-78.5533, -31.2085)
  line L120 (-78.5533, -31.2085) -> (-78.7943, -31.92)
  spline S119 degree 2 poles (-78.7943, -31.92) (-78.8449, -32.0678) (-78.7049, -32.2738) (-78.5533, -32.2738) knots 0 0 0 1 2 2 2
  line L121 (-78.5533, -32.2738) -> (-77.3091, -32.2738)
  spline S120 degree 2 poles (-77.3091, -32.2738) (-77.1303, -32.2738) (-77.1925, -32.4527) knots 0 0 0 1 1 1
  spline S121 degree 2 poles (-77.1925, -32.4527) (-77.2508, -32.6276) (-77.4296, -32.6276) knots 0 0 0 1 1 1
  line L122 (-77.4296, -32.6276) -> (-78.6738, -32.6276)
  spline S122 degree 2 poles (-78.6738, -32.6276) (-78.9693, -32.6276) (-79.2454, -32.2077) (-79.1482, -31.9161) knots 0 0 0 1 2 2 2
  line L123 (-79.1482, -31.9161) -> (-77.939, -28.3625)
  line L124 (-77.5852, -28.3625) -> (-78.4328, -30.8547)
  line L125 (-78.4328, -30.8547) -> (-77.3636, -30.8547)
  spline S123 degree 2 poles (-77.3636, -30.8547) (-77.2119, -30.8547) (-76.932, -30.6447) (-76.8814, -30.497) knots 0 0 0 1 2 2 2
  line L126 (-76.8814, -30.497) -> (-76.1544, -28.3625)
  spline S124 degree 2 poles (-76.1544, -28.3625) (-76.1038, -28.2147) (-76.2438, -28.0048) (-76.3954, -28.0048) knots 0 0 0 1 2 2 2
  line L127 (-76.3954, -28.0048) -> (-77.1031, -28.0048)
  spline S125 degree 2 poles (-77.1031, -28.0048) (-77.2547, -28.0048) (-77.5346, -28.2147) (-77.5852, -28.3625) knots 0 0 0 1 2 2 2
  spline S126 degree 2 poles (-80.6062, -27.8298) (-80.544, -27.651) (-80.3651, -27.651) knots 0 0 0 1 1 1
  line L128 (-80.3651, -27.651) -> (-79.1171, -27.651)
  spline S127 degree 2 poles (-79.1171, -27.651) (-78.8216, -27.651) (-78.5455, -28.067) (-78.6466, -28.3625) knots 0 0 0 1 2 2 2
  line L129 (-78.6466, -28.3625) -> (-79.5525, -31.0297)
  spline S128 degree 2 poles (-79.5525, -31.0297) (-79.6147, -31.2085) (-79.7897, -31.2085) knots 0 0 0 1 1 1
  spline S129 degree 2 poles (-79.7897, -31.2085) (-79.9685, -31.2085) (-79.9063, -31.0297) knots 0 0 0 1 1 1
  line L130 (-79.9063, -31.0297) -> (-79.0004, -28.3625)
  spline S130 degree 2 poles (-79.0004, -28.3625) (-78.9499, -28.2147) (-79.0898, -28.0048) (-79.2376, -28.0048) knots 0 0 0 1 2 2 2
  line L131 (-79.2376, -28.0048) -> (-80.3107, -28.0048)
  line L132 (-80.3107, -28.0048) -> (-81.3371, -31.0297)
  spline S131 degree 2 poles (-81.3371, -31.0297) (-81.3993, -31.2085) (-81.5743, -31.2085) knots 0 0 0 1 1 1
  spline S132 degree 2 poles (-81.5743, -31.2085) (-81.7531, -31.2085) (-81.6909, -31.0297) knots 0 0 0 1 1 1
  line L133 (-81.6909, -31.0297) -> (-80.6062, -27.8298)
  spline S133 degree 2 poles (-83.4483, -27.8298) (-83.3861, -27.651) (-83.2111, -27.651) knots 0 0 0 1 1 1
  spline S134 degree 2 poles (-83.2111, -27.651) (-83.0323, -27.651) (-83.0945, -27.8298) knots 0 0 0 1 1 1
  line L134 (-83.0945, -27.8298) -> (-84.1209, -30.8547)
  line L135 (-84.1209, -30.8547) -> (-83.3744, -30.8547)
  line L136 (-83.3744, -30.8547) -> (-81.652, -27.7909)
  spline S135 degree 2 poles (-81.652, -27.7909) (-81.5743, -27.651) (-81.4343, -27.651) knots 0 0 0 1 1 1
  spline S136 degree 2 poles (-81.4343, -27.651) (-81.2555, -27.651) (-81.3138, -27.822) knots 0 0 0 1 1 1
  spline S137 degree 2 poles (-81.3138, -27.822) (-81.3216, -27.8415) (-81.3332, -27.8687) knots 0 0 0 1 1 1
  line L137 (-81.3332, -27.8687) -> (-83.1295, -31.0685)
  spline S138 degree 2 poles (-83.1295, -31.0685) (-83.2111, -31.2085) (-83.3511, -31.2085) knots 0 0 0 1 1 1
  line L138 (-83.3511, -31.2085) -> (-84.4164, -31.2085)
  spline S139 degree 2 poles (-84.4164, -31.2085) (-84.5953, -31.2085) (-84.5331, -31.0297) knots 0 0 0 1 1 1
  line L139 (-84.5331, -31.0297) -> (-83.4483, -27.8298)
  spline S140 degree 2 poles (-86.6209, -27.8259) (-86.5587, -27.6393) (-86.3838, -27.6393) knots 0 0 0 1 1 1
  spline S141 degree 2 poles (-86.3838, -27.6393) (-86.2321, -27.6393) (-86.0961, -27.8881) knots 0 0 0 1 1 1
  spline S142 degree 2 poles (-86.0961, -27.8881) (-85.8045, -27.651) (-85.4817, -27.651) knots 0 0 0 1 1 1
  line L140 (-85.4817, -27.651) -> (-84.7702, -27.651)
  spline S143 degree 2 poles (-84.7702, -27.651) (-84.4747, -27.651) (-84.1987, -28.067) (-84.2998, -28.3625) knots 0 0 0 1 2 2 2
  line L141 (-84.2998, -28.3625) -> (-85.0268, -30.497)
  spline S144 degree 2 poles (-85.0268, -30.497) (-85.124, -30.7886) (-85.6878, -31.2085) (-85.9794, -31.2085) knots 0 0 0 1 2 2 2
  line L142 (-85.9794, -31.2085) -> (-87.2236, -31.2085)
  spline S145 degree 2 poles (-87.2236, -31.2085) (-87.4024, -31.2085) (-87.3402, -31.0297) knots 0 0 0 1 1 1
  line L143 (-87.3402, -31.0297) -> (-86.4343, -28.3547)
  spline S146 degree 2 poles (-86.4343, -28.3547) (-86.341, -28.0864) (-86.551, -27.9931) knots 0 0 0 1 1 1
  spline S147 degree 2 poles (-86.551, -27.9931) (-86.6637, -27.9426) (-86.6209, -27.8259) knots 0 0 0 1 1 1
  line L144 (-86.0805, -28.3625) -> (-86.9281, -30.8547)
  line L145 (-86.9281, -30.8547) -> (-85.8589, -30.8547)
  spline S148 degree 2 poles (-85.8589, -30.8547) (-85.7111, -30.8547) (-85.4312, -30.6447) (-85.3807, -30.497) knots 0 0 0 1 2 2 2
  line L146 (-85.3807, -30.497) -> (-84.6536, -28.3625)
  spline S149 degree 2 poles (-84.6536, -28.3625) (-84.6031, -28.2147) (-84.743, -28.0048) (-84.8908, -28.0048) knots 0 0 0 1 2 2 2
  line L147 (-84.8908, -28.0048) -> (-85.6023, -28.0048)
  spline S150 degree 2 poles (-85.6023, -28.0048) (-85.75, -28.0048) (-86.03, -28.2147) (-86.0805, -28.3625) knots 0 0 0 1 2 2 2
  point P0 (0, 0)
  dimension "d3" = 294
  dimension "d4" = 90
  constraints: 2 other
emboss "Рельеф1" sketch "Эскиз9" operation cut depth 1 direction (0, -1, 0)
sketch "Эскиз10" plane through (0, 2, 0) normal (0, 1, 0) x (1, 0, 0)
  circle A0 centre (87, -36) radius 1.5
  circle A1 centre (57, -36) radius 1.5
  circle A2 centre (-112, -15) radius 1.5
  circle A3 centre (-132, -15) radius 1.5
  circle A4 centre (-112, 15) radius 1.5
  circle A5 centre (-132, 15) radius 1.5
  line L0 (-147, -45) -> (147, -45) projected
  line L1 (147, -45) -> (147, 42) projected
  line L2 (-147, 42) -> (-147, -45) projected
  line L3 (144, 45) -> (-144, 45) projected
  point P0 (0, 0)
  dimension "d42" = 3
  dimension "d43" = 9
  dimension "d44" = 9
  dimension "d45" = 30
  dimension "d46" = 60
  dimension "d47" = 20
  dimension "d48" = 15
  dimension "d49" = 20
  dimension "d50" = 30
  dimension "d51" = 30
  dimension "d52" = 15
  dimension "d53" = 30
  dimension "d54" = 30
  constraints: 6 centre point, 5 equal radius
  measures "d42" diameter of A0
  measures "d43" distance from line of L0 A0.centre
  measures "d44" distance from line of L0 A1.centre
  measures "d45" distance of A1.centre A0.centre
  measures "d46" distance from line of L1 A0.centre
  measures "d47" distance of A2.centre A3.centre
  measures "d48" distance from line of L2 A3.centre
  measures "d49" distance of A5.centre A4.centre
  measures "d50" distance of A2.centre A4.centre
  measures "d51" distance from line of L3 A4.centre
  measures "d52" distance from line of L2 A5.centre
  measures "d53" distance of A3.centre A5.centre
  measures "d54" distance from line of L3 A5.centre
extrude "Выдавливание9" cut sketch "Эскиз10" against normal up to next
sketch "Эскиз11" plane through (-147, -2, 45) normal (-1, 0, 0) x (0, 0, 1)
  line L0 (-87, 0) -> (-87, 4) projected
  line L1 (0, 0) -> (-87, 0) projected
  line L2 (0, 0) -> (0, 4) projected
  line L3 (-87, 4) -> (0, 4) projected
  line L4 (-87, 4) -> (-90, 4) projected
  line L5 (-90, 4) -> (-90, 0) projected
  line L6 (-90, 0) -> (-87, 0) projected
  line L7 (-87, 0) -> (-87, 4) projected
  line L8 (-21, -50) -> (-21, 0) projected
  line L9 (-21, 0) -> (-21, 4)
  line L10 (-87, 4) -> (0, 4) projected
  point P0 (-45, 2)
  point P1 (-21, 4)
  constraints: 2 end point, 1 perpendicular, 1 point on line
extrude "Выдавливание10" cut sketch "Эскиз11" against normal blind 4 contours L6 L5 L4 L0 | L0 L3 L9 L1
sketch "Эскиз12" plane through (0, 2, 0) normal (0, 1, 0) x (1, 0, 0)
  line L0 (-143, 25) -> (-143, 15) projected
  line L1 (-147, 25) -> (-143, 25) projected
  line L2 (-147, 15) -> (-147, 25) projected
  line L3 (-147, 15) -> (-143, 15) projected
  line L4 (-143, -4) -> (-143, -14) projected
  line L5 (-147, -4) -> (-143, -4) projected
  line L6 (-147, -14) -> (-147, -4) projected
  line L7 (-147, -14) -> (-143, -14) projected
  point P0 (0, 0)
extrude "Выдавливание11" add sketch "Эскиз12" against normal blind 4
mirror "Зеркальное отражение3" about plane through (0, 0, 0) normal (1, 0, 0) of "Выдавливание10", "Выдавливание11"
sketch "Эскиз13" plane through (0, 2, 0) normal (0, 1, 0) x (1, 0, 0)
  line L0 (-143, 15) -> (-143, -4) projected
  line L1 (-143, -4) -> (-143, 15) projected
  line L2 (-143, 6.95) -> (-133, 6.95)
  line L3 (-133, 6.95) -> (-133, 4.05)
  line L4 (-133, 4.05) -> (-143, 4.05)
  line L5 (-143, 4.05) -> (-143, 6.95)
  line L6 (-135.7, 8.4) -> (-138, 8.4)
  line L7 (-138, 8.4) -> (-138, 2.6)
  line L8 (-138, 2.6) -> (-135.7, 2.6)
  line L9 (-135.7, 2.6) -> (-135.7, 8.4)
  line L10 (-133, 5.5) -> (-143, 5.5) construction
  line L11 (-143, 25) -> (-143, 45) projected
  line L12 (-143, 36.45) -> (-133, 36.45)
  line L13 (-133, 36.45) -> (-133, 33.55)
  line L14 (-133, 33.55) -> (-143, 33.55)
  line L15 (-143, 33.55) -> (-143, 36.45)
  line L16 (-135.7, 37.9) -> (-138, 37.9)
  line L17 (-138, 37.9) -> (-138, 32.1)
  line L18 (-138, 32.1) -> (-135.7, 32.1)
  line L19 (-135.7, 32.1) -> (-135.7, 37.9)
  line L20 (-133, 35) -> (-143, 35) construction
  point P0 (0, 0)
  point P1 (-135.7, 5.5)
  point P2 (-138, 6.95)
  point P3 (-143, 4.05)
  point P4 (-138, 4.05)
  point P5 (-135.7, 4.05)
  point P6 (-135.7, 6.95)
  point P7 (-135.7, 35)
  point P8 (-138, 36.45)
  point P9 (-138, 33.55)
  point P10 (-135.7, 33.55)
  point P11 (-135.7, 36.45)
  dimension "d61" = 10
  dimension "d62" = 2.9
  dimension "d63" = 2.3
  dimension "d64" = 5.8
  dimension "d65" = 5
  dimension "d68" = 5
  constraints: 36 end point, 8 midpoint, 8 parallel, 5 horizontal, 4 equal length, 4 perpendicular, 4 point on line
  measures "d61" distance of L3.end L4.end
  measures "d62" distance of L2.end L3.end
  measures "d63" distance of L7.end L8.end
  measures "d64" distance of L8.end L6.start
  measures "d65" distance between parallel lines of L0 L7
  measures "d68" distance between parallel lines of L11 L17
extrude "Выдавливание12" cut sketch "Эскиз13" against normal up to next
mirror "Зеркальное отражение4" about plane through (0, 0, 0) normal (1, 0, 0) of "Выдавливание12"
